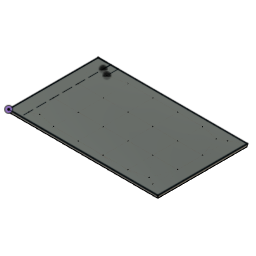
CNCTable (Autodesk Fusion 360 archive; units mm, degrees)
design "CNCTable" references "autodesk 3ax table head xyz"
Autodesk Fusion 360 part; units mm, degrees
sketch "Sketch4" plane through (0, 0, 0) normal (0, 0, 1) x (1, 0, 0)
  line L0 (0, 0) -> (300, 0)
  line L1 (300, 0) -> (300, 180)
  line L2 (300, 180) -> (0, 180)
  line L3 (0, 180) -> (0, 0)
  line L4 (0, 180) -> (25, 180) construction
  line L5 (25, 180) -> (25, 0) construction
  line L6 (25, 180) -> (25, 165) construction
  line L7 (0, 180) -> (40, 180) construction
  line L8 (40, 180) -> (40, 157.5) construction
  dimension "d50" = 300
  dimension "d51" = 180
  dimension "d52" = 25
  dimension "d53" = 15
  dimension "d54" = 40
  dimension "d72" = 22.5
  constraint horizontal L0
  constraint vertical L1
  constraint horizontal L2
  constraint vertical L3
  constraint coincident L0.start L3.end
  constraint perpendicular L3 L4
  constraint coincident L0 L5.end
  constraint perpendicular L0 L5
  constraint perpendicular L4 L6
  constraint perpendicular L3 L7
  constraint perpendicular L2 L8
  measures "d50" distance of L0.start L0.end
  measures "d51" distance of L0.start L2.end
  measures "d52" distance of L2.end L4.end
  measures "d53" distance of L4.end L6.end
  measures "d54" distance of L2.end L7.end
  measures "d72" distance of L7.end L8.end
extrude "Extrude4" add sketch "Sketch4" against normal blind 5
hole "Hole4" at (25, 165, 0) direction (0, 0, -1) diameter 1 depth 5 tip angle 180
pattern_linear "R-Pattern4" count 6 spacing 50 along (1, 0, 0) count 4 spacing 50 along (0, -1, 0) of "Hole4"
hole "Hole6" at (40, 157.5, 0) direction (0, 0, -1) diameter 1 depth 5 tip angle 180
pattern_linear "R-Pattern5" count 2 spacing 220 along (1, 0, 0) count 2 spacing 135 along (0, -1, 0) of "Hole6"
equation "d53 = ( ( 180 - 150 ) / 2 ) * 1 mm"
equation "d72 = ( 180 mm - 135 mm ) / 2"
